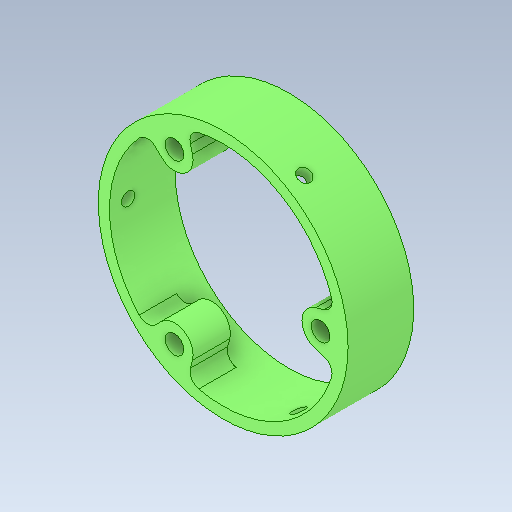
# Autodesk Inventor part: Board Spacer
Saved by Autodesk Inventor 2020 (Build 240168000, 168)
## iProperties
Created: 2018-03-06
Part Number: Board Spacer
Material: Generic
Document SubType Name: Modeling
Designer: Alex
Density: 1 g/cm^3
Appearance: Default
Description: 3D Printed Space for Power Supply and Filament Board
Vendor: n/a
Author: Alex
Autodesk Inventor part; units mm, degrees
ref_plane "YZ Plane" through (0, 0, 0) normal (1, 0, 0) x (0, 1, 0)
ref_plane "XZ Plane" through (0, 0, 0) normal (0, 1, 0) x (-1, 0, 0)
ref_plane "XY Plane" through (0, 0, 0) normal (0, 0, 1) x (1, 0, 0)
sketch "Sketch1" plane through (0, 0, 0) normal (0, 0, 1) x (1, 0, 0)
  circle A0 centre (0, 0) radius 19.3675
  circle A1 centre (0, 0) radius 21.2725
  dimension "d0" = 38.735
  dimension "d1" = 42.545
  constraints: 2 centre point, 2 coincident
  measures "d0" diameter of A0
  measures "d1" diameter of A1
extrude "Extrusion1" add sketch "Sketch1" along normal blind 6.35
sketch "Sketch2" plane through (0, 0, 0) normal (0, 0, -1) x (-1, 0, 0)
  line L0 (-16.5947, 0) -> (8.2973, 14.3714) construction
  line L1 (8.2973, 14.3714) -> (8.2973, -14.3714) construction
  line L2 (8.2973, -14.3714) -> (-16.5947, 0) construction
  arc A0 (-15.7729, -3.0668) -> (-15.7729, 3.0668) centre (-16.5947, 0) ccw
  circle A1 centre (0, 0) radius 19.3675 construction
  arc A2 (-18.9661, 3.9224) -> (-18.9661, -3.9224) centre (0, 0) ccw
  line L3 (-15.7729, -3.0668) -> (-18.9661, -3.9224)
  line L4 (-15.7729, 3.0668) -> (-18.9661, 3.9224)
  line L5 (0, 0) -> (-17.8049, 0) construction
  arc A3 (10.5424, -12.1263) -> (5.2305, -15.1932) centre (8.2973, -14.3714) ccw
  arc A4 (6.0861, -18.3864) -> (12.88, -14.4639) centre (0, 0) ccw
  line L6 (10.5424, -12.1263) -> (12.88, -14.4639)
  line L7 (5.2305, -15.1932) -> (6.0861, -18.3864)
  arc A5 (5.2305, 15.1932) -> (10.5424, 12.1263) centre (8.2973, 14.3714) ccw
  arc A6 (12.88, 14.4639) -> (6.0861, 18.3864) centre (0, 0) ccw
  line L8 (5.2305, 15.1932) -> (6.0861, 18.3864)
  line L9 (10.5424, 12.1263) -> (12.88, 14.4639)
  line L10 (0, 0) -> (-13.4197, 0) construction
  circle A7 centre (0, 0) radius 19.05 construction
  line L11 (19.05, -19.05) -> (-19.05, -19.05) construction
  line L12 (-19.05, -19.05) -> (-19.05, 19.05) construction
  line L13 (-19.05, 19.05) -> (19.05, 19.05) construction
  line L14 (19.05, 19.05) -> (19.05, -19.05) construction
  line L15 (19.05, -19.05) -> (-19.05, 19.05) construction
  line L16 (-19.05, -19.05) -> (19.05, 19.05) construction
  point P0 (8.9024, -15.4195)
  point P1 (8.9024, 15.4195)
  point P2 (0, 19.05)
  dimension "d62" = 38.1
  dimension "d5" = 6.35
  dimension "d7" = 30
  dimension "d10" = 360
  dimension "d59" = 13.4197
  dimension "d63" = 38.1
  dimension "d65" = 24.892
  constraints: 37 end point, 21 point on circle, 6 centre point, 6 coincident, 3 midpoint, 2 horizontal, 2 parallel, 1 equal length, 1 horizontal alignment, 1 perpendicular, 1 point on line, 1 tangent, 1 vertical alignment, 47 other
  measures "d5" diameter of A0
  measures "d7" angle of L3 L4
  measures "d59" distance of L10.start L10.end
  measures "d63" distance of L12.end L13.end
  measures "d65" distance from line of L0.start L1
extrude "Extrusion2" add sketch "Sketch2" against normal up to surface (6.35 mm away)
fillet "Fillet1" radius 1.905 6 edges at (-6.0861, 18.3864, 3.175) (-12.88, 14.4639, 3.175) (18.9661, -3.9224, 3.175) (18.9661, 3.9224, 3.175) (-12.88, -14.4639, 3.175) (-6.0861, -18.3864, 3.175)
sketch "Sketch3" plane through (0, 0, 6.35) normal (0, 0, 1) x (1, 0, 0)
  arc A0 (-10.5424, 12.1263) -> (-5.2305, 15.1932) centre (-8.2973, 14.3714) ccw construction
  arc A1 (-5.2305, -15.1932) -> (-10.5424, -12.1263) centre (-8.2973, -14.3714) ccw construction
  arc A2 (15.7729, 3.0668) -> (15.7729, -3.0668) centre (16.5947, 0) ccw construction
  point P0 (0, 0)
hole "Hole1" at (-8.2973, 14.3714, 6.35) at (16.5947, 0, 6.35) at (-8.2973, -14.3714, 6.35) direction (0, 0, -1) diameter 3.175 end through all
sketch "Sketch11" plane through (0, 0, 0) normal (1, 0, 0) x (0, 1, 0)
  circle A0 centre (0, 3.175) radius 1.1303
  line L0 (13.0654, 0) -> (-13.0654, 0) projected
  line L1 (-13.0654, 6.35) -> (13.0654, 6.35) projected
  point P0 (0, 0)
  point P1 (0, 0)
  dimension "d51" = 2.2606
  dimension "d52" = 3.175
  dimension "d53" = 6.35
  constraints: 1 centre point, 1 midpoint, 1 vertical alignment
  measures "d51" diameter of A0
  measures "d52" distance of point (0, 0) A0.centre
  measures "d53" distance between parallel lines of L0 L1
extrude "Extrusion7" cut sketch "Sketch11" against normal through all
pattern_circular "Circular Pattern1" count 3 over 360 about axis through (0, 0, 0) along (0, 0, 1) of "Extrusion7"
sketch "Sketch12" plane through (0, 0, 0) normal (0, 0, -1) x (-1, 0, 0)
  arc A0 (4.1667, 18.914) -> (-18.4633, 5.8486) centre (0, 0) ccw projected
  circle A1 centre (0, 0) radius 19.3675
  circle A2 centre (0, 0) radius 21.2725
  constraints: 2 coincident, 1 centre point, 3 other
extrude "Extrusion8" add sketch "Sketch12" along normal blind 4.826
equation "\"d52\" = 0.5 * d53"
body "Solid1"
